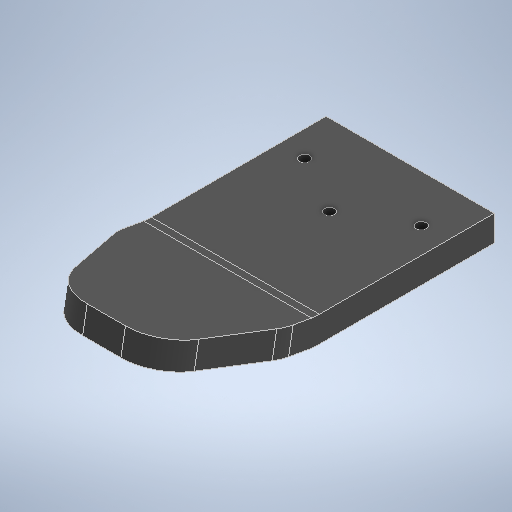
# Autodesk Inventor part: toe_sole_front
Saved by Autodesk Inventor 2026.1 (Build 301233020, 233B)
## iProperties
Created: 2024-02-12
Part Number: toe_sole_front
Material: 一般
Document SubType Name: モデリング
Designer: hibik
Density: 1 g/cm^3
Appearance: 既定
Sheet Metal Rule: Default
Author: hibik
Autodesk Inventor part; units mm, degrees
ref_plane "YZ Plane" through (0, 0, 0) normal (1, 0, 0) x (0, 1, 0)
ref_plane "XZ Plane" through (0, 0, 0) normal (0, 1, 0) x (-1, 0, 0)
ref_plane "XY Plane" through (0, 0, 0) normal (0, 0, 1) x (1, 0, 0)
sketch "スケッチ1" plane through (0, 0, 0) normal (0, 1, 0) x (-1, 0, 0)
  line L0 (26, 0) -> (0, 0)
  line L1 (0, 0) -> (0, -15)
  line L2 (0, -15) -> (26, -15)
  line L3 (26, -15) -> (26, 0)
  line L4 (36.4849, 5.9511) -> (26, -20)
  line L5 (26, -20) -> (0, -20)
  line L6 (0, -20) -> (-10.4849, 5.9511)
  arc A0 (36.4849, 5.9511) -> (-10.4849, 5.9511) centre (13, -20) ccw
  line L7 (0, 0) -> (26, -15)
  line L8 (0, -15) -> (26, 0)
  line L9 (4, -2.3077) -> (22, -2.3077)
  line L10 (22, -2.3077) -> (22, -12.6923)
  line L11 (22, -12.6923) -> (4, -12.6923)
  line L12 (4, -12.6923) -> (4, -2.3077)
  circle A1 centre (4, -2.3077) radius 0.8
  circle A2 centre (4, -12.6923) radius 0.8
  circle A3 centre (22, -2.3077) radius 0.8
  circle A4 centre (22, -12.6923) radius 0.8
  circle A5 centre (13, -7.5) radius 0.8
  line L13 (38, 8) -> (-12, 8)
  line L14 (-12, 8) -> (-12, -20)
  line L15 (-12, -20) -> (38, -20)
  line L16 (38, -20) -> (38, 8)
  point P0 (22.6929, -13.0921)
  point P1 (21.2, -12.6923)
  point P2 (13, 8)
  point P3 (13, -7.5)
  point P4 (34, 8)
  point P5 (0, -20)
  point P6 (-8, 8)
  point P7 (0, -20)
  dimension "d0" = 26
  dimension "d1" = 15
  dimension "d4" = 22
  dimension "d5" = 22
  dimension "d6" = 5
  dimension "d7" = 35
  dimension "d23" = 4
  dimension "d24" = 1.6
  dimension "d25" = 1.6
  dimension "d26" = 1.6
  dimension "d27" = 1.6
  dimension "d32" = 1.6
  dimension "d54" = 50
  dimension "d55" = 28
  constraints: 34 end point, 6 centre point, 6 coincident, 6 parallel, 5 point on line, 4 horizontal, 4 midpoint, 3 perpendicular, 2 point on circle, 1 collinear, 1 vertical alignment
  measures "d0" distance of L0.start L0.end
  measures "d1" distance of L2.end L0.start
  measures "d4" angle of L3 L4
  measures "d5" angle of L6 L1
  measures "d6" distance between parallel lines of L5 L2
  measures "d7" radius of A0
  measures "d23" distance between parallel lines of L1 L12
  measures "d24" diameter of A1
  measures "d25" diameter of A2
  measures "d26" diameter of A3
  measures "d27" diameter of A4
  measures "d32" diameter of A5
  measures "d54" distance of L13.start L13.end
  measures "d55" distance of L13.end L14.end
extrude "押し出し1" add sketch "スケッチ1" along normal blind 1.5 contours L8 A3 L9 A1 L7 L0 | L3 L7 A4 L10 A3 L8 | L7 A1 L12 A2 L8 L1 | L2 L8 A2 L11 A4 L7 | A3 L10 L8 | L8 L9 A3 | A1 L9 L7 | L7 L12 A1 | L10 A3 L8 | L8 A3 L9 | A3 L8 A5 L7 A1 L9 | L9 A1 L7 | L7 A1 L12 | A1 L7 A5 L8 A2 L12 | L11 A2 L8 A5 L7 A4 | A3 L10 A4 L7 A5 L8 | A0 L13 L16 L15 L4 | L4 L5 L6 A0 L13 | L15 L14 L13 A0 L6
sketch "スケッチ5" plane through (0, 0, 0) normal (0, -1, 0) x (1, 0, 0)
  line L0 (12, -20) -> (-38, -20) projected
  line L1 (12, 8) -> (12, -20) projected
  line L2 (-38, 8) -> (12, 8) projected
  line L3 (-38, -20) -> (-38, 8) projected
  circle A0 centre (-13, -7.5) radius 2.5
  circle A1 centre (-4, -12.6923) radius 2.5
  circle A2 centre (-22, -12.6923) radius 2.5
  line L4 (10, 9) -> (2, 9)
  line L5 (2, 9) -> (2, -21)
  line L6 (2, -21) -> (10, -21)
  line L7 (10, -21) -> (10, 9)
  line L8 (-28, 9) -> (-36, 9)
  line L9 (-36, 9) -> (-36, -21)
  line L10 (-36, -21) -> (-28, -21)
  line L11 (-28, -21) -> (-28, 9)
  point P0 (0, 0)
  point P1 (10, -6)
  point P2 (12, -6)
  point P3 (-28, -6)
  dimension "d56" = 5
  dimension "d57" = 5
  dimension "d58" = 5
  dimension "d61" = 8
  dimension "d62" = 30
  dimension "d63" = 2
  dimension "d64" = 2
  constraints: 16 end point, 4 parallel, 3 centre point, 3 midpoint, 2 equal length, 2 horizontal, 2 horizontal alignment, 2 perpendicular
  measures "d56" diameter of A0
  measures "d57" diameter of A1
  measures "d58" diameter of A2
  measures "d61" distance of L6.end L5.end
  measures "d62" distance of L5.end L4.end
  measures "d63" distance between parallel lines of L1 L7
  measures "d64" distance between parallel lines of L3 L9
extrude "押し出し5" add sketch "スケッチ5" along normal blind 2.5 contours L0 L7 L2 L1 | L0 L11 L2 L5 | L0 L3 L2 L9
fillet "フィレット3" radius 1 4 edges at (10, -2.5, -6) (2, -2.5, -6) (-28, -2.5, -6) (-36, -2.5, -6)
sketch "スケッチ6" plane through (0, -2.5, 0) normal (0, -1, 0) x (1, 0, 0)
  line L0 (-38, -20) -> (12, -20) projected
  line L1 (-26, -20) -> (0, -20)
  line L2 (0, -20) -> (0, 8)
  line L3 (0, 8) -> (-26, 8)
  line L4 (-26, 8) -> (-26, -20)
  line L5 (1, 8) -> (1, -20) projected
  line L6 (-27, -20) -> (-27, 8) projected
  line L7 (12, 8) -> (-38, 8) projected
  line L8 (-38, 8) -> (-38, -20) projected
  line L9 (12, -20) -> (12, 8) projected
  point P0 (0, 0)
  point P1 (1, 10)
  point P2 (1, -18.5)
  point P3 (-27, -18.5)
  point P4 (-27, 10)
  point P5 (-26, 8)
  point P6 (0, 8)
  point P7 (0, -20)
  dimension "d66" = 1
  dimension "d67" = 1
  constraints: 8 end point, 2 parallel, 1 collinear, 1 horizontal, 1 perpendicular, 1 point on line
  measures "d66" distance between parallel lines of L5 L2
  measures "d67" distance between parallel lines of L6 L4
extrude "押し出し6" cut sketch "スケッチ6" against normal through all contours L8 L7 L6 L0 | L6 L7 L4 L0 | L2 L7 L5 L0 | L5 L7 L9 L0
sketch "スケッチ7" plane through (0, -2.5, 8) normal (1, 0, 0) x (0, 0, -1)
  line L0 (0, 0) -> (0, 4) projected
  line L1 (0, 0) -> (-19.6962, 3.473)
  line L2 (-19.6962, 3.473) -> (-19.0016, 7.4122)
  line L3 (-19.0016, 7.4122) -> (0.35, 4)
  line L4 (0, 4) -> (28, 4) projected
  line L5 (28, 0) -> (0, 0) projected
  point P0 (8, 2.5)
  point P1 (7, 4)
  point P2 (7, 0)
  dimension "d70" = 10
  dimension "d71" = 20
  constraints: 6 end point, 2 perpendicular, 1 equal length, 1 point on line
  measures "d70" angle of L5 L1
  measures "d71" distance from line of L0.start L2
extrude "押し出し7" add sketch "スケッチ7" against normal up to surface (26 mm away)
chamfer "面取り2" distance 15 distance2 5 1 edges at (0, 2.9426, 27.3489) measured on face at (0, 2.8558, 26.8565)
chamfer "面取り3" distance 15 distance2 5 1 edges at (-26, 2.9426, 27.3489) measured on face at (-26, 2.8558, 26.8565)
fillet "フィレット4" radius 7 6 edges at (0, 0.3379, 12.5767) (-5, 2.9426, 27.3489) (-21, 2.9426, 27.3489) (-26, 0.3379, 12.5767) (-13, -2.5, 8) (-13, 1.5, 7.65)
sketch "スケッチ9" plane through (0, -2.5, 0) normal (0, -1, 0) x (1, 0, 0)
  line L0 (-9.7144, 0.766) -> (-11, -0.766)
  line L1 (-11, -0.766) -> (-3.3396, -7.1939)
  line L2 (-3.3396, -7.1939) -> (-2.054, -5.6618)
  line L3 (-2.054, -5.6618) -> (-9.7144, 0.766)
  line L4 (-31.2, 0) -> (5.2, 0) construction
  line L5 (-26, 0) -> (0, 0) construction
  line L6 (-26, 7.3876) -> (-26, -20) projected
  line L7 (0, -20) -> (0, 7.3876) projected
  line L8 (-9.7144, 5.766) -> (-11, 4.234)
  line L9 (-2.054, -0.6618) -> (-9.7144, 5.766)
  line L10 (-3.3396, -2.1939) -> (-2.054, -0.6618)
  line L11 (-11, 4.234) -> (-3.3396, -2.1939)
  line L12 (-9.7144, 10.766) -> (-11, 9.234)
  line L13 (-2.054, 4.3382) -> (-9.7144, 10.766)
  line L14 (-3.3396, 2.8061) -> (-2.054, 4.3382)
  line L15 (-11, 9.234) -> (-3.3396, 2.8061)
  line L16 (-26, 7.3876) -> (0, 7.3876) projected
  line L17 (-13, 0) -> (-13, 7.3876)
  line L18 (-16.2856, 0.766) -> (-15, -0.766)
  line L19 (-15, -0.766) -> (-22.6604, -7.1939)
  line L20 (-22.6604, -7.1939) -> (-23.946, -5.6618)
  line L21 (-23.946, -5.6618) -> (-16.2856, 0.766)
  line L22 (-16.2856, 5.766) -> (-15, 4.234)
  line L23 (-23.946, -0.6618) -> (-16.2856, 5.766)
  line L24 (-22.6604, -2.1939) -> (-23.946, -0.6618)
  line L25 (-15, 4.234) -> (-22.6604, -2.1939)
  line L26 (-16.2856, 10.766) -> (-15, 9.234)
  line L27 (-23.946, 4.3382) -> (-16.2856, 10.766)
  line L28 (-22.6604, 2.8061) -> (-23.946, 4.3382)
  line L29 (-15, 9.234) -> (-22.6604, 2.8061)
  point P0 (0, 0)
  point P1 (5.2, 0)
  point P2 (-10.3572, 0)
  point P3 (-10.3572, 5)
  point P4 (-10.3572, 10)
  point P5 (-26, 0)
  point P6 (-15.6428, 0)
  point P7 (-15.6428, 5)
  point P8 (-15.6428, 10)
  point P9 (-5.6881, 7.3876)
  point P10 (-8.7996, 7.3876)
  point P11 (-17.2004, 7.3876)
  point P12 (-20.3119, 7.3876)
  dimension "d81" = 40
  dimension "d82" = 2
  dimension "d83" = 2
  dimension "d84" = 10
  dimension "d87" = 5
  constraints: 52 end point, 17 symmetric about line, 3 midpoint, 2 parallel, 2 point on line, 1 horizontal, 1 perpendicular, 1 vertical, 21 other
  measures "d81" angle to the sketch x axis of L1
  measures "d82" horizontal distance of L0.end L17.start
  measures "d83" distance between parallel lines of L1 L3
  measures "d84" distance between parallel lines of L2 L0
  measures "d87" distance of L0.start L8.start
extrude "押し出し8" cut sketch "スケッチ9" against normal blind 0.8
sketch "スケッチ10" plane through (-15.9547, 0.973, 27.6962) normal (0, -0.9848078, 0.1736482) x (1, 0, 0)
  line L0 (6.2403, -9.4276) -> (4.9547, -10.9597)
  line L1 (4.9547, -10.9597) -> (12.6151, -17.3876)
  line L2 (12.6151, -17.3876) -> (13.9007, -15.8555)
  line L3 (13.9007, -15.8555) -> (6.2403, -9.4276)
  line L4 (-15.2453, -27.4443) -> (21.1547, -27.4443) projected
  line L5 (15.9547, -19.3876) -> (8.8179, -19.3876) projected
  line L6 (15.9547, -57.4957) -> (15.9547, 10.3807) projected
  line L7 (13.9007, -10.8555) -> (6.2403, -4.4276)
  line L8 (6.2403, -4.4276) -> (4.9547, -5.9597)
  line L9 (4.9547, -5.9597) -> (12.6151, -12.3876)
  line L10 (12.6151, -12.3876) -> (13.9007, -10.8555)
  line L11 (2.9547, -27.8785) -> (2.9547, -20.6031) projected
  line L12 (-0.3309, -9.4276) -> (0.9547, -10.9597)
  line L13 (0.9547, -10.9597) -> (-6.7058, -17.3876)
  line L14 (-6.7058, -17.3876) -> (-7.9913, -15.8555)
  line L15 (-7.9913, -15.8555) -> (-0.3309, -9.4276)
  line L16 (-7.9913, -10.8555) -> (-0.3309, -4.4276)
  line L17 (-0.3309, -4.4276) -> (0.9547, -5.9597)
  line L18 (0.9547, -5.9597) -> (-6.7058, -12.3876)
  line L19 (-6.7058, -12.3876) -> (-7.9913, -10.8555)
  point P0 (15.9547, -27.4443)
  point P1 (4.9547, -18.747)
  point P2 (13.9007, -23.6062)
  dimension "d94" = 40
  dimension "d95" = 2
  dimension "d96" = 2
  dimension "d99" = 5
  constraints: 32 end point, 8 symmetric about line, 2 parallel, 2 vertical alignment, 1 perpendicular, 1 vertical, 8 other
  measures "d94" angle of L4 L1
  measures "d95" distance between parallel lines of L3 L1
  measures "d96" distance from line of L5 L1.end
  measures "d99" distance of L2.end L7.start
extrude "押し出し9" cut sketch "スケッチ10" against normal blind 0.8
equation "\"d5\" = d4"
equation "\"BendRadius\" = Thickness"
equation "\"BendReliefWidth\" = Thickness"
equation "\"BendReliefDepth\" = 0.5 * Thickness"
equation "\"CornerReliefSize\" = 4 * Thickness"
equation "\"MinimumRemnant\" = 2 * Thickness"
equation "\"TransitionRadius\" = BendRadius"
equation "\"JacobiRadiusSize\" = BendRadius"
equation "\"GapSize\" = Thickness"
equation "\"Thickness\" = 3.048"
